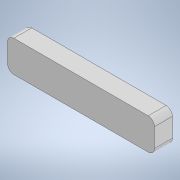
# Autodesk Inventor part: tococo
Saved by Autodesk Inventor 2022 (Build 260153000, 153)
## iProperties
Created: 2022-08-08
Part Number: tococo
Material: Genérico
Document SubType Name: Modeling
Designer: JK
Density: 1 g/cm^3
Appearance: Valor por defecto
Author: JK
Autodesk Inventor part; units mm, degrees
ref_plane "YZ Plane" through (0, 0, 0) normal (1, 0, 0) x (0, 1, 0)
ref_plane "XZ Plane" through (0, 0, 0) normal (0, 1, 0) x (-1, 0, 0)
ref_plane "XY Plane" through (0, 0, 0) normal (0, 0, 1) x (1, 0, 0)
sketch "Boceto1" plane through (0, 0, 0) normal (0, 1, 0) x (-1, 0, 0)
  line L0 (-23.35, 2.85) -> (23.35, 2.85)
  line L1 (23.35, 2.85) -> (23.35, -2.85)
  line L2 (23.35, -2.85) -> (-23.35, -2.85)
  line L3 (-23.35, -2.85) -> (-23.35, 2.85)
  line L4 (-23.35, 2.85) -> (23.35, -2.85) construction
  line L5 (23.35, 2.85) -> (-23.35, -2.85) construction
  point P0 (0, 0)
  dimension "d0" = 5.7
  dimension "d1" = 46.7
  constraints: 12 end point, 2 midpoint, 2 parallel, 1 horizontal, 1 perpendicular
  measures "d0" distance between parallel lines of L2 L0
  measures "d1" distance of L0.start L0.end
extrude "Extrusión1" add sketch "Boceto1" along normal blind 10
fillet "Empalme1" radius 2 4 edges at (-23.35, 0, 0) (-23.35, 10, 0) (23.35, 0, 0) (23.35, 10, 0)
